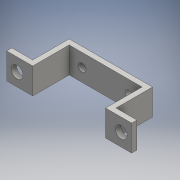
# Autodesk Inventor part: EncoderBracket
Saved by Autodesk Inventor 2016 (Build 200138000, 138)
## iProperties
Created: 2015-06-06
Part Number: EncoderBracket
Material: Generic
Document SubType Name: Modeling
Designer: Erin
Density: 1 g/cm^3
Appearance: Default
Author: Erin
Autodesk Inventor part; units mm, degrees
ref_plane "YZ Plane" through (0, 0, 0) normal (1, 0, 0) x (0, 1, 0)
ref_plane "XZ Plane" through (0, 0, 0) normal (0, 1, 0) x (-1, 0, 0)
ref_plane "XY Plane" through (0, 0, 0) normal (0, 0, 1) x (1, 0, 0)
sketch "Sketch1" plane through (0, 0, 0) normal (0, 0, 1) x (1, 0, 0)
  line L0 (-16, 19.8024) -> (16, 19.8024)
  line L1 (16, 19.8024) -> (16, 17.8024)
  line L2 (16, 17.8024) -> (-16, 17.8024)
  line L3 (-16, 17.8024) -> (-16, 19.8024)
  line L4 (-16, 17.8024) -> (-14, 17.8024)
  line L5 (-14, 17.8024) -> (-14, 5.8024)
  line L6 (-14, 5.8024) -> (-16, 5.8024)
  line L7 (-16, 5.8024) -> (-16, 17.8024)
  line L8 (16, 17.8024) -> (14, 17.8024)
  line L9 (14, 17.8024) -> (14, 5.8024)
  line L10 (14, 5.8024) -> (16, 5.8024)
  line L11 (16, 5.8024) -> (16, 17.8024)
  line L12 (-14, 5.8024) -> (-24, 5.8024)
  line L13 (-24, 5.8024) -> (-24, 3.8024)
  line L14 (-24, 3.8024) -> (-14, 3.8024)
  line L15 (-14, 3.8024) -> (-14, 5.8024)
  line L16 (14, 5.8024) -> (24, 5.8024)
  line L17 (24, 5.8024) -> (24, 3.8024)
  line L18 (24, 3.8024) -> (14, 3.8024)
  line L19 (14, 3.8024) -> (14, 5.8024)
  point P0 (0, 0)
  point P1 (0, 19.8024)
  dimension "d0" = 32
  dimension "d1" = 2
  dimension "d2" = 2
  dimension "d3" = 12
  dimension "d4" = 2
  dimension "d5" = 12
  dimension "d6" = 10
  dimension "d7" = 2
  dimension "d8" = 10
  dimension "d9" = 2
  constraints: 40 end point, 10 parallel, 5 horizontal, 5 perpendicular, 1 midpoint, 1 vertical alignment
  measures "d0" distance of L1.end L2.end
  measures "d1" distance of L0.end L1.end
  measures "d2" distance of L5.end L6.end
  measures "d3" distance of L4.end L5.end
  measures "d4" distance of L10.end L9.end
  measures "d5" distance of L9.end L8.end
  measures "d6" distance of L14.end L13.end
  measures "d7" distance of L13.end L12.end
  measures "d8" distance of L17.end L18.end
  measures "d9" distance of L16.end L17.end
extrude "Extrusion1" add sketch "Sketch1" along normal blind 10
sketch "Sketch2" plane through (-16, 19.8024, 0) normal (0, 1, 0) x (1, 0, 0)
  line L0 (32, 0) -> (0, 0) projected
  line L1 (0, 0) -> (0, -10) projected
  line L2 (32, -10) -> (0, -10) projected
  line L3 (32, 0) -> (32, -10) projected
  line L4 (0, 0) -> (0, -10) projected
  line L5 (32, 0) -> (32, -10) projected
  circle A0 centre (7, -5) radius 1.5
  circle A1 centre (25, -5) radius 1.5
  line L6 (2, -10) -> (30, -10) projected
  line L7 (16, -10) -> (16, 0) construction
  dimension "d12" = 3
  dimension "d13" = 3
  dimension "d14" = 9
  dimension "d15" = 9
  constraints: 2 centre point, 2 end point, 1 midpoint, 1 vertical
  measures "d12" diameter of A0
  measures "d13" diameter of A1
  measures "d14" distance from line of A0.centre L7
  measures "d15" distance from line of A1.centre L7
extrude "Extrusion2" cut sketch "Sketch2" against normal blind 3 contours A0 | A1
sketch "Sketch3" plane through (-24, 5.8024, 0) normal (0, 1, 0) x (1, 0, 0)
  line L0 (8, -10) -> (8, 0) projected
  line L1 (8, 0) -> (0, 0) projected
  line L2 (0, 0) -> (0, -10) projected
  line L3 (8, -10) -> (0, -10) projected
  circle A0 centre (4, -5) radius 2.25
  point P0 (24, 0)
  dimension "d18" = 4.5
  constraints: 1 centre point
  measures "d18" diameter of A0
extrude "Extrusion3" cut sketch "Sketch3" against normal blind 3 contours A0
mirror "Mirror1" about plane through (0, 0, 0) normal (1, 0, 0) of "Extrusion3"
sketch "Sketch4" plane through (14, 3.8024, 0) normal (0, -1, 0) x (1, 0, 0)
  circle A0 centre (6, 5) radius 2.25 projected
  line L0 (0, 0) -> (10, 0) projected
  line L1 (10, 0) -> (10, 10) projected
  line L2 (0, 10) -> (10, 10) projected
  line L3 (0, 0) -> (0, 10) projected
  circle A1 centre (-34, 5) radius 2.25 projected
  line L4 (-38, 0) -> (-28, 0) projected
  line L5 (-28, 0) -> (-28, 10) projected
  line L6 (-38, 10) -> (-28, 10) projected
  line L7 (-38, 0) -> (-38, 10) projected
  point P0 (-14, 0)
  dimension "d21" = 40
  measures "d21" distance of A1.centre A0.centre
body "Solid1"
